Autodesk Inventor part; units mm, degrees
(part 3 of 5)
sketch "Block4" plane through (0, 0, 0) normal (0, 0, 1) x (1, 0, 0)
  line L0 (2.525, -1.7375) -> (2.525, 11.2625)
  line L1 (16.525, -1.7375) -> (16.525, 11.2625)
  line L2 (3.025, -2.2375) -> (16.025, -2.2375)
  line L3 (3.025, 11.7625) -> (16.025, 11.7625)
  arc A0 (2.525, -1.7375) -> (3.025, -2.2375) centre (3.025, -1.7375) ccw
  arc A1 (3.025, 11.7625) -> (2.525, 11.2625) centre (3.025, 11.2625) ccw
  arc A2 (16.025, -2.2375) -> (16.525, -1.7375) centre (16.025, -1.7375) ccw
  arc A3 (16.525, 11.2625) -> (16.025, 11.7625) centre (16.025, 11.2625) ccw
  line L4 (2.525, 36.3625) -> (2.525, 49.3625)
  line L5 (16.525, 36.3625) -> (16.525, 49.3625)
  line L6 (3.025, 35.8625) -> (16.025, 35.8625)
  line L7 (3.025, 49.8625) -> (16.025, 49.8625)
  arc A4 (2.525, 36.3625) -> (3.025, 35.8625) centre (3.025, 36.3625) ccw
  arc A5 (3.025, 49.8625) -> (2.525, 49.3625) centre (3.025, 49.3625) ccw
  arc A6 (16.025, 35.8625) -> (16.525, 36.3625) centre (16.025, 36.3625) ccw
  arc A7 (16.525, 49.3625) -> (16.025, 49.8625) centre (16.025, 49.3625) ccw
  line L8 (2.525, 55.4125) -> (2.525, 68.4125)
  line L9 (16.525, 55.4125) -> (16.525, 68.4125)
  line L10 (3.025, 54.9125) -> (16.025, 54.9125)
  line L11 (3.025, 68.9125) -> (16.025, 68.9125)
  arc A8 (2.525, 55.4125) -> (3.025, 54.9125) centre (3.025, 55.4125) ccw
  arc A9 (3.025, 68.9125) -> (2.525, 68.4125) centre (3.025, 68.4125) ccw
  arc A10 (16.025, 54.9125) -> (16.525, 55.4125) centre (16.025, 55.4125) ccw
  arc A11 (16.525, 68.4125) -> (16.025, 68.9125) centre (16.025, 68.4125) ccw
  line L12 (2.525, 74.4625) -> (2.525, 87.4625)
  line L13 (16.525, 74.4625) -> (16.525, 87.4625)
  line L14 (3.025, 73.9625) -> (16.025, 73.9625)
  line L15 (3.025, 87.9625) -> (16.025, 87.9625)
  arc A12 (2.525, 74.4625) -> (3.025, 73.9625) centre (3.025, 74.4625) ccw
  arc A13 (3.025, 87.9625) -> (2.525, 87.4625) centre (3.025, 87.4625) ccw
  arc A14 (16.025, 73.9625) -> (16.525, 74.4625) centre (16.025, 74.4625) ccw
  arc A15 (16.525, 87.4625) -> (16.025, 87.9625) centre (16.025, 87.4625) ccw
  line L16 (2.525, 93.5125) -> (2.525, 106.5125)
  line L17 (16.525, 93.5125) -> (16.525, 106.5125)
  line L18 (3.025, 93.0125) -> (16.025, 93.0125)
  line L19 (3.025, 107.0125) -> (16.025, 107.0125)
  arc A16 (2.525, 93.5125) -> (3.025, 93.0125) centre (3.025, 93.5125) ccw
  arc A17 (3.025, 107.0125) -> (2.525, 106.5125) centre (3.025, 106.5125) ccw
  arc A18 (16.025, 93.0125) -> (16.525, 93.5125) centre (16.025, 93.5125) ccw
  arc A19 (16.525, 106.5125) -> (16.025, 107.0125) centre (16.025, 106.5125) ccw
  line L20 (2.525, 122.0875) -> (2.525, 135.0875)
  line L21 (16.525, 122.0875) -> (16.525, 135.0875)
  line L22 (3.025, 121.5875) -> (16.025, 121.5875)
  line L23 (3.025, 135.5875) -> (16.025, 135.5875)
  arc A20 (2.525, 122.0875) -> (3.025, 121.5875) centre (3.025, 122.0875) ccw
  arc A21 (3.025, 135.5875) -> (2.525, 135.0875) centre (3.025, 135.0875) ccw
  arc A22 (16.025, 121.5875) -> (16.525, 122.0875) centre (16.025, 122.0875) ccw
  arc A23 (16.525, 135.0875) -> (16.025, 135.5875) centre (16.025, 135.0875) ccw
  line L24 (2.525, 141.1375) -> (2.525, 154.1375)
  line L25 (16.525, 141.1375) -> (16.525, 154.1375)
  line L26 (3.025, 140.6375) -> (16.025, 140.6375)
  line L27 (3.025, 154.6375) -> (16.025, 154.6375)
  arc A24 (2.525, 141.1375) -> (3.025, 140.6375) centre (3.025, 141.1375) ccw
  arc A25 (3.025, 154.6375) -> (2.525, 154.1375) centre (3.025, 154.1375) ccw
  arc A26 (16.025, 140.6375) -> (16.525, 141.1375) centre (16.025, 141.1375) ccw
  arc A27 (16.525, 154.1375) -> (16.025, 154.6375) centre (16.025, 154.1375) ccw
  line L28 (2.525, 160.1875) -> (2.525, 173.1875)
  line L29 (16.525, 160.1875) -> (16.525, 173.1875)
  line L30 (3.025, 159.6875) -> (16.025, 159.6875)
  line L31 (3.025, 173.6875) -> (16.025, 173.6875)
  arc A28 (2.525, 160.1875) -> (3.025, 159.6875) centre (3.025, 160.1875) ccw
  arc A29 (3.025, 173.6875) -> (2.525, 173.1875) centre (3.025, 173.1875) ccw
  arc A30 (16.025, 159.6875) -> (16.525, 160.1875) centre (16.025, 160.1875) ccw
  arc A31 (16.525, 173.1875) -> (16.025, 173.6875) centre (16.025, 173.1875) ccw
  line L32 (2.525, 179.2375) -> (2.525, 192.2375)
  line L33 (16.525, 179.2375) -> (16.525, 192.2375)
  line L34 (3.025, 178.7375) -> (16.025, 178.7375)
  line L35 (3.025, 192.7375) -> (16.025, 192.7375)
  arc A32 (2.525, 179.2375) -> (3.025, 178.7375) centre (3.025, 179.2375) ccw
  arc A33 (3.025, 192.7375) -> (2.525, 192.2375) centre (3.025, 192.2375) ccw
  arc A34 (16.025, 178.7375) -> (16.525, 179.2375) centre (16.025, 179.2375) ccw
  arc A35 (16.525, 192.2375) -> (16.025, 192.7375) centre (16.025, 192.2375) ccw
  line L36 (2.525, 207.8125) -> (2.525, 220.8125)
  line L37 (16.525, 207.8125) -> (16.525, 220.8125)
  line L38 (3.025, 207.3125) -> (16.025, 207.3125)
  line L39 (3.025, 221.3125) -> (16.025, 221.3125)
  arc A36 (2.525, 207.8125) -> (3.025, 207.3125) centre (3.025, 207.8125) ccw
  arc A37 (3.025, 221.3125) -> (2.525, 220.8125) centre (3.025, 220.8125) ccw
  arc A38 (16.025, 207.3125) -> (16.525, 207.8125) centre (16.025, 207.8125) ccw
  arc A39 (16.525, 220.8125) -> (16.025, 221.3125) centre (16.025, 220.8125) ccw
  line L40 (2.525, 226.8625) -> (2.525, 239.8625)
  line L41 (16.525, 226.8625) -> (16.525, 239.8625)
  line L42 (3.025, 226.3625) -> (16.025, 226.3625)
  line L43 (3.025, 240.3625) -> (16.025, 240.3625)
  arc A40 (2.525, 226.8625) -> (3.025, 226.3625) centre (3.025, 226.8625) ccw
  arc A41 (3.025, 240.3625) -> (2.525, 239.8625) centre (3.025, 239.8625) ccw
  arc A42 (16.025, 226.3625) -> (16.525, 226.8625) centre (16.025, 226.8625) ccw
  arc A43 (16.525, 239.8625) -> (16.025, 240.3625) centre (16.025, 239.8625) ccw
  line L44 (2.525, 245.9125) -> (2.525, 258.9125)
  line L45 (16.525, 245.9125) -> (16.525, 258.9125)
  line L46 (3.025, 245.4125) -> (16.025, 245.4125)
  line L47 (3.025, 259.4125) -> (16.025, 259.4125)
  arc A44 (2.525, 245.9125) -> (3.025, 245.4125) centre (3.025, 245.9125) ccw
  arc A45 (3.025, 259.4125) -> (2.525, 258.9125) centre (3.025, 258.9125) ccw
  arc A46 (16.025, 245.4125) -> (16.525, 245.9125) centre (16.025, 245.9125) ccw
  arc A47 (16.525, 258.9125) -> (16.025, 259.4125) centre (16.025, 258.9125) ccw
  line L48 (2.525, 264.9625) -> (2.525, 277.9625)
  line L49 (16.525, 264.9625) -> (16.525, 277.9625)
  line L50 (3.025, 264.4625) -> (16.025, 264.4625)
  line L51 (3.025, 278.4625) -> (16.025, 278.4625)
  arc A48 (2.525, 264.9625) -> (3.025, 264.4625) centre (3.025, 264.9625) ccw
  arc A49 (3.025, 278.4625) -> (2.525, 277.9625) centre (3.025, 277.9625) ccw
  arc A50 (16.025, 264.4625) -> (16.525, 264.9625) centre (16.025, 264.9625) ccw
  arc A51 (16.525, 277.9625) -> (16.025, 278.4625) centre (16.025, 277.9625) ccw
  line L52 (26.3375, -1.7375) -> (26.3375, 11.2625)
  line L53 (40.3375, -1.7375) -> (40.3375, 11.2625)
  line L54 (26.8375, -2.2375) -> (39.8375, -2.2375)
  line L55 (26.8375, 11.7625) -> (39.8375, 11.7625)
  arc A52 (26.3375, -1.7375) -> (26.8375, -2.2375) centre (26.8375, -1.7375) ccw
  arc A53 (26.8375, 11.7625) -> (26.3375, 11.2625) centre (26.8375, 11.2625) ccw
  arc A54 (39.8375, -2.2375) -> (40.3375, -1.7375) centre (39.8375, -1.7375) ccw
  arc A55 (40.3375, 11.2625) -> (39.8375, 11.7625) centre (39.8375, 11.2625) ccw
  line L56 (26.3375, 17.3125) -> (26.3375, 30.3125)
  line L57 (40.3375, 17.3125) -> (40.3375, 30.3125)
  line L58 (26.8375, 16.8125) -> (39.8375, 16.8125)
  line L59 (26.8375, 30.8125) -> (39.8375, 30.8125)
  arc A56 (26.3375, 17.3125) -> (26.8375, 16.8125) centre (26.8375, 17.3125) ccw
  arc A57 (26.8375, 30.8125) -> (26.3375, 30.3125) centre (26.8375, 30.3125) ccw
  arc A58 (39.8375, 16.8125) -> (40.3375, 17.3125) centre (39.8375, 17.3125) ccw
  arc A59 (40.3375, 30.3125) -> (39.8375, 30.8125) centre (39.8375, 30.3125) ccw
  line L60 (26.3375, 36.3625) -> (26.3375, 49.3625)
  line L61 (40.3375, 36.3625) -> (40.3375, 49.3625)
  line L62 (26.8375, 35.8625) -> (39.8375, 35.8625)
  line L63 (26.8375, 49.8625) -> (39.8375, 49.8625)
  arc A60 (26.3375, 36.3625) -> (26.8375, 35.8625) centre (26.8375, 36.3625) ccw
  arc A61 (26.8375, 49.8625) -> (26.3375, 49.3625) centre (26.8375, 49.3625) ccw
  arc A62 (39.8375, 35.8625) -> (40.3375, 36.3625) centre (39.8375, 36.3625) ccw
  arc A63 (40.3375, 49.3625) -> (39.8375, 49.8625) centre (39.8375, 49.3625) ccw
  line L64 (26.3375, 55.4125) -> (26.3375, 68.4125)
  line L65 (40.3375, 55.4125) -> (40.3375, 68.4125)
  line L66 (26.8375, 54.9125) -> (39.8375, 54.9125)
  line L67 (26.8375, 68.9125) -> (39.8375, 68.9125)
  arc A64 (26.3375, 55.4125) -> (26.8375, 54.9125) centre (26.8375, 55.4125) ccw
  arc A65 (26.8375, 68.9125) -> (26.3375, 68.4125) centre (26.8375, 68.4125) ccw
  arc A66 (39.8375, 54.9125) -> (40.3375, 55.4125) centre (39.8375, 55.4125) ccw
  arc A67 (40.3375, 68.4125) -> (39.8375, 68.9125) centre (39.8375, 68.4125) ccw
  line L68 (26.3375, 74.4625) -> (26.3375, 87.4625)
  line L69 (40.3375, 74.4625) -> (40.3375, 87.4625)
  line L70 (26.8375, 73.9625) -> (39.8375, 73.9625)
  line L71 (26.8375, 87.9625) -> (39.8375, 87.9625)
  arc A68 (26.3375, 74.4625) -> (26.8375, 73.9625) centre (26.8375, 74.4625) ccw
  arc A69 (26.8375, 87.9625) -> (26.3375, 87.4625) centre (26.8375, 87.4625) ccw
  arc A70 (39.8375, 73.9625) -> (40.3375, 74.4625) centre (39.8375, 74.4625) ccw
  arc A71 (40.3375, 87.4625) -> (39.8375, 87.9625) centre (39.8375, 87.4625) ccw
  line L72 (26.3375, 93.5125) -> (26.3375, 106.5125)
  line L73 (40.3375, 93.5125) -> (40.3375, 106.5125)
  line L74 (26.8375, 93.0125) -> (39.8375, 93.0125)
  line L75 (26.8375, 107.0125) -> (39.8375, 107.0125)
  arc A72 (26.3375, 93.5125) -> (26.8375, 93.0125) centre (26.8375, 93.5125) ccw
  arc A73 (26.8375, 107.0125) -> (26.3375, 106.5125) centre (26.8375, 106.5125) ccw
  arc A74 (39.8375, 93.0125) -> (40.3375, 93.5125) centre (39.8375, 93.5125) ccw
  arc A75 (40.3375, 106.5125) -> (39.8375, 107.0125) centre (39.8375, 106.5125) ccw
  line L76 (26.3375, 112.5625) -> (26.3375, 125.5625)
  line L77 (40.3375, 112.5625) -> (40.3375, 125.5625)
  line L78 (26.8375, 112.0625) -> (39.8375, 112.0625)
  line L79 (26.8375, 126.0625) -> (39.8375, 126.0625)
  arc A76 (26.3375, 112.5625) -> (26.8375, 112.0625) centre (26.8375, 112.5625) ccw
  arc A77 (26.8375, 126.0625) -> (26.3375, 125.5625) centre (26.8375, 125.5625) ccw
  arc A78 (39.8375, 112.0625) -> (40.3375, 112.5625) centre (39.8375, 112.5625) ccw
  arc A79 (40.3375, 125.5625) -> (39.8375, 126.0625) centre (39.8375, 125.5625) ccw
  line L80 (26.3375, 131.6125) -> (26.3375, 144.6125)
  line L81 (40.3375, 131.6125) -> (40.3375, 144.6125)
  line L82 (26.8375, 131.1125) -> (39.8375, 131.1125)
  line L83 (26.8375, 145.1125) -> (39.8375, 145.1125)
  arc A80 (26.3375, 131.6125) -> (26.8375, 131.1125) centre (26.8375, 131.6125) ccw
  arc A81 (26.8375, 145.1125) -> (26.3375, 144.6125) centre (26.8375, 144.6125) ccw
  arc A82 (39.8375, 131.1125) -> (40.3375, 131.6125) centre (39.8375, 131.6125) ccw
  arc A83 (40.3375, 144.6125) -> (39.8375, 145.1125) centre (39.8375, 144.6125) ccw
  line L84 (26.3375, 150.6625) -> (26.3375, 163.6625)
  line L85 (40.3375, 150.6625) -> (40.3375, 163.6625)
  line L86 (26.8375, 150.1625) -> (39.8375, 150.1625)
  line L87 (26.8375, 164.1625) -> (39.8375, 164.1625)
  arc A84 (26.3375, 150.6625) -> (26.8375, 150.1625) centre (26.8375, 150.6625) ccw
  arc A85 (26.8375, 164.1625) -> (26.3375, 163.6625) centre (26.8375, 163.6625) ccw
  arc A86 (39.8375, 150.1625) -> (40.3375, 150.6625) centre (39.8375, 150.6625) ccw
  arc A87 (40.3375, 163.6625) -> (39.8375, 164.1625) centre (39.8375, 163.6625) ccw
  line L88 (26.3375, 169.7125) -> (26.3375, 182.7125)
  line L89 (40.3375, 169.7125) -> (40.3375, 182.7125)
  line L90 (26.8375, 169.2125) -> (39.8375, 169.2125)
  line L91 (26.8375, 183.2125) -> (39.8375, 183.2125)
  arc A88 (26.3375, 169.7125) -> (26.8375, 169.2125) centre (26.8375, 169.7125) ccw
  arc A89 (26.8375, 183.2125) -> (26.3375, 182.7125) centre (26.8375, 182.7125) ccw
  arc A90 (39.8375, 169.2125) -> (40.3375, 169.7125) centre (39.8375, 169.7125) ccw
  arc A91 (40.3375, 182.7125) -> (39.8375, 183.2125) centre (39.8375, 182.7125) ccw
  line L92 (26.3375, 188.7625) -> (26.3375, 201.7625)
  line L93 (40.3375, 188.7625) -> (40.3375, 201.7625)
  line L94 (26.8375, 188.2625) -> (39.8375, 188.2625)
  line L95 (26.8375, 202.2625) -> (39.8375, 202.2625)
  arc A92 (26.3375, 188.7625) -> (26.8375, 188.2625) centre (26.8375, 188.7625) ccw
  arc A93 (26.8375, 202.2625) -> (26.3375, 201.7625) centre (26.8375, 201.7625) ccw
  arc A94 (39.8375, 188.2625) -> (40.3375, 188.7625) centre (39.8375, 188.7625) ccw
  arc A95 (40.3375, 201.7625) -> (39.8375, 202.2625) centre (39.8375, 201.7625) ccw
  line L96 (26.3375, 207.8125) -> (26.3375, 220.8125)
  line L97 (40.3375, 207.8125) -> (40.3375, 220.8125)
  line L98 (26.8375, 207.3125) -> (39.8375, 207.3125)
  line L99 (26.8375, 221.3125) -> (39.8375, 221.3125)
  arc A96 (26.3375, 207.8125) -> (26.8375, 207.3125) centre (26.8375, 207.8125) ccw
  arc A97 (26.8375, 221.3125) -> (26.3375, 220.8125) centre (26.8375, 220.8125) ccw
  arc A98 (39.8375, 207.3125) -> (40.3375, 207.8125) centre (39.8375, 207.8125) ccw
  arc A99 (40.3375, 220.8125) -> (39.8375, 221.3125) centre (39.8375, 220.8125) ccw
  line L100 (26.3375, 226.8625) -> (26.3375, 239.8625)
  line L101 (40.3375, 226.8625) -> (40.3375, 239.8625)
  line L102 (26.8375, 226.3625) -> (39.8375, 226.3625)
  line L103 (26.8375, 240.3625) -> (39.8375, 240.3625)
  arc A100 (26.3375, 226.8625) -> (26.8375, 226.3625) centre (26.8375, 226.8625) ccw
  arc A101 (26.8375, 240.3625) -> (26.3375, 239.8625) centre (26.8375, 239.8625) ccw
  arc A102 (39.8375, 226.3625) -> (40.3375, 226.8625) centre (39.8375, 226.8625) ccw
  arc A103 (40.3375, 239.8625) -> (39.8375, 240.3625) centre (39.8375, 239.8625) ccw
  line L104 (26.3375, 255.4375) -> (26.3375, 268.4375)
  line L105 (40.3375, 255.4375) -> (40.3375, 268.4375)
  line L106 (26.8375, 254.9375) -> (39.8375, 254.9375)
  line L107 (26.8375, 268.9375) -> (39.8375, 268.9375)
  arc A104 (26.3375, 255.4375) -> (26.8375, 254.9375) centre (26.8375, 255.4375) ccw
  arc A105 (26.8375, 268.9375) -> (26.3375, 268.4375) centre (26.8375, 268.4375) ccw
  arc A106 (39.8375, 254.9375) -> (40.3375, 255.4375) centre (39.8375, 255.4375) ccw
  arc A107 (40.3375, 268.4375) -> (39.8375, 268.9375) centre (39.8375, 268.4375) ccw
  line L108 (27.3375, 246.9995) -> (27.3375, 252.9995)
  line L109 (42.3375, 246.9995) -> (42.3375, 252.9995)
  line L110 (27.8375, 246.4995) -> (41.8375, 246.4995)
  line L111 (27.8375, 253.4995) -> (41.8375, 253.4995)
  arc A108 (27.3375, 246.9995) -> (27.8375, 246.4995) centre (27.8375, 246.9995) ccw
  arc A109 (27.8375, 253.4995) -> (27.3375, 252.9995) centre (27.8375, 252.9995) ccw
  arc A110 (41.8375, 246.4995) -> (42.3375, 246.9995) centre (41.8375, 246.9995) ccw
  arc A111 (42.3375, 252.9995) -> (41.8375, 253.4995) centre (41.8375, 252.9995) ccw
  line L112 (27.3375, 270.8755) -> (27.3375, 276.8755)
  line L113 (42.3375, 270.8755) -> (42.3375, 276.8755)
  line L114 (27.8375, 270.3755) -> (41.8375, 270.3755)
  line L115 (27.8375, 277.3755) -> (41.8375, 277.3755)
  arc A112 (27.3375, 270.8755) -> (27.8375, 270.3755) centre (27.8375, 270.8755) ccw
  arc A113 (27.8375, 277.3755) -> (27.3375, 276.8755) centre (27.8375, 276.8755) ccw
  arc A114 (41.8375, 270.3755) -> (42.3375, 270.8755) centre (41.8375, 270.8755) ccw
  arc A115 (42.3375, 276.8755) -> (41.8375, 277.3755) centre (41.8375, 276.8755) ccw
  line L116 (26.3375, 288.775) -> (26.3375, 301.775)
  line L117 (40.3375, 288.775) -> (40.3375, 301.775)
  line L118 (26.8375, 288.275) -> (39.8375, 288.275)
  line L119 (26.8375, 302.275) -> (39.8375, 302.275)
  arc A116 (26.3375, 288.775) -> (26.8375, 288.275) centre (26.8375, 288.775) ccw
  arc A117 (26.8375, 302.275) -> (26.3375, 301.775) centre (26.8375, 301.775) ccw
  arc A118 (39.8375, 288.275) -> (40.3375, 288.775) centre (39.8375, 288.775) ccw
  arc A119 (40.3375, 301.775) -> (39.8375, 302.275) centre (39.8375, 301.775) ccw
  line L120 (26.3375, 307.825) -> (26.3375, 320.825)
  line L121 (40.3375, 307.825) -> (40.3375, 320.825)
  line L122 (26.8375, 307.325) -> (39.8375, 307.325)
  line L123 (26.8375, 321.325) -> (39.8375, 321.325)
  arc A120 (26.3375, 307.825) -> (26.8375, 307.325) centre (26.8375, 307.825) ccw
  arc A121 (26.8375, 321.325) -> (26.3375, 320.825) centre (26.8375, 320.825) ccw
  arc A122 (39.8375, 307.325) -> (40.3375, 307.825) centre (39.8375, 307.825) ccw
  arc A123 (40.3375, 320.825) -> (39.8375, 321.325) centre (39.8375, 320.825) ccw
  line L124 (26.3375, 326.875) -> (26.3375, 339.875)
  line L125 (40.3375, 326.875) -> (40.3375, 339.875)
  line L126 (26.8375, 326.375) -> (39.8375, 326.375)
  line L127 (26.8375, 340.375) -> (39.8375, 340.375)
  arc A124 (26.3375, 326.875) -> (26.8375, 326.375) centre (26.8375, 326.875) ccw
  arc A125 (26.8375, 340.375) -> (26.3375, 339.875) centre (26.8375, 339.875) ccw
  arc A126 (39.8375, 326.375) -> (40.3375, 326.875) centre (39.8375, 326.875) ccw
  arc A127 (40.3375, 339.875) -> (39.8375, 340.375) centre (39.8375, 339.875) ccw
  line L128 (45.3875, 3.025) -> (45.3875, 16.025)
  line L129 (59.3875, 3.025) -> (59.3875, 16.025)
  line L130 (45.8875, 2.525) -> (58.8875, 2.525)
  line L131 (45.8875, 16.525) -> (58.8875, 16.525)
  arc A128 (45.3875, 3.025) -> (45.8875, 2.525) centre (45.8875, 3.025) ccw
  arc A129 (45.8875, 16.525) -> (45.3875, 16.025) centre (45.8875, 16.025) ccw
  arc A130 (58.8875, 2.525) -> (59.3875, 3.025) centre (58.8875, 3.025) ccw
  arc A131 (59.3875, 16.025) -> (58.8875, 16.525) centre (58.8875, 16.025) ccw
  line L132 (45.3875, 26.8375) -> (45.3875, 39.8375)
  line L133 (59.3875, 26.8375) -> (59.3875, 39.8375)
  line L134 (45.8875, 26.3375) -> (58.8875, 26.3375)
  line L135 (45.8875, 40.3375) -> (58.8875, 40.3375)
  arc A132 (45.3875, 26.8375) -> (45.8875, 26.3375) centre (45.8875, 26.8375) ccw
  arc A133 (45.8875, 40.3375) -> (45.3875, 39.8375) centre (45.8875, 39.8375) ccw
  arc A134 (58.8875, 26.3375) -> (59.3875, 26.8375) centre (58.8875, 26.8375) ccw
  arc A135 (59.3875, 39.8375) -> (58.8875, 40.3375) centre (58.8875, 39.8375) ccw
  line L136 (45.3875, 45.8875) -> (45.3875, 58.8875)
  line L137 (59.3875, 45.8875) -> (59.3875, 58.8875)
  line L138 (45.8875, 45.3875) -> (58.8875, 45.3875)
  line L139 (45.8875, 59.3875) -> (58.8875, 59.3875)
  arc A136 (45.3875, 45.8875) -> (45.8875, 45.3875) centre (45.8875, 45.8875) ccw
  arc A137 (45.8875, 59.3875) -> (45.3875, 58.8875) centre (45.8875, 58.8875) ccw
  arc A138 (58.8875, 45.3875) -> (59.3875, 45.8875) centre (58.8875, 45.8875) ccw
  arc A139 (59.3875, 58.8875) -> (58.8875, 59.3875) centre (58.8875, 58.8875) ccw
  line L140 (45.3875, 64.9375) -> (45.3875, 77.9375)
  line L141 (59.3875, 64.9375) -> (59.3875, 77.9375)
  line L142 (45.8875, 64.4375) -> (58.8875, 64.4375)
  line L143 (45.8875, 78.4375) -> (58.8875, 78.4375)
  arc A140 (45.3875, 64.9375) -> (45.8875, 64.4375) centre (45.8875, 64.9375) ccw
  arc A141 (45.8875, 78.4375) -> (45.3875, 77.9375) centre (45.8875, 77.9375) ccw
  arc A142 (58.8875, 64.4375) -> (59.3875, 64.9375) centre (58.8875, 64.9375) ccw
  arc A143 (59.3875, 77.9375) -> (58.8875, 78.4375) centre (58.8875, 77.9375) ccw
  line L144 (45.3875, 83.9875) -> (45.3875, 96.9875)
  line L145 (59.3875, 83.9875) -> (59.3875, 96.9875)
  line L146 (45.8875, 83.4875) -> (58.8875, 83.4875)
  line L147 (45.8875, 97.4875) -> (58.8875, 97.4875)
  arc A144 (45.3875, 83.9875) -> (45.8875, 83.4875) centre (45.8875, 83.9875) ccw
  arc A145 (45.8875, 97.4875) -> (45.3875, 96.9875) centre (45.8875, 96.9875) ccw
  arc A146 (58.8875, 83.4875) -> (59.3875, 83.9875) centre (58.8875, 83.9875) ccw
  arc A147 (59.3875, 96.9875) -> (58.8875, 97.4875) centre (58.8875, 96.9875) ccw
  line L148 (45.3875, 103.0375) -> (45.3875, 116.0375)
  line L149 (59.3875, 103.0375) -> (59.3875, 116.0375)
  line L150 (45.8875, 102.5375) -> (58.8875, 102.5375)
  line L151 (45.8875, 116.5375) -> (58.8875, 116.5375)
  arc A148 (45.3875, 103.0375) -> (45.8875, 102.5375) centre (45.8875, 103.0375) ccw
  arc A149 (45.8875, 116.5375) -> (45.3875, 116.0375) centre (45.8875, 116.0375) ccw
  arc A150 (58.8875, 102.5375) -> (59.3875, 103.0375) centre (58.8875, 103.0375) ccw
  arc A151 (59.3875, 116.0375) -> (58.8875, 116.5375) centre (58.8875, 116.0375) ccw
  line L152 (45.3875, 122.0875) -> (45.3875, 135.0875)
  line L153 (59.3875, 122.0875) -> (59.3875, 135.0875)
  line L154 (45.8875, 121.5875) -> (58.8875, 121.5875)
  line L155 (45.8875, 135.5875) -> (58.8875, 135.5875)
  arc A152 (45.3875, 122.0875) -> (45.8875, 121.5875) centre (45.8875, 122.0875) ccw
  arc A153 (45.8875, 135.5875) -> (45.3875, 135.0875) centre (45.8875, 135.0875) ccw
  arc A154 (58.8875, 121.5875) -> (59.3875, 122.0875) centre (58.8875, 122.0875) ccw
  arc A155 (59.3875, 135.0875) -> (58.8875, 135.5875) centre (58.8875, 135.0875) ccw
  line L156 (45.3875, 141.1375) -> (45.3875, 154.1375)
  line L157 (59.3875, 141.1375) -> (59.3875, 154.1375)
  line L158 (45.8875, 140.6375) -> (58.8875, 140.6375)
  line L159 (45.8875, 154.6375) -> (58.8875, 154.6375)
  arc A156 (45.3875, 141.1375) -> (45.8875, 140.6375) centre (45.8875, 141.1375) ccw
  arc A157 (45.8875, 154.6375) -> (45.3875, 154.1375) centre (45.8875, 154.1375) ccw
  arc A158 (58.8875, 140.6375) -> (59.3875, 141.1375) centre (58.8875, 141.1375) ccw
  arc A159 (59.3875, 154.1375) -> (58.8875, 154.6375) centre (58.8875, 154.1375) ccw
  line L160 (45.3875, 160.1875) -> (45.3875, 173.1875)
  line L161 (59.3875, 160.1875) -> (59.3875, 173.1875)
  line L162 (45.8875, 159.6875) -> (58.8875, 159.6875)
  line L163 (45.8875, 173.6875) -> (58.8875, 173.6875)
  arc A160 (45.3875, 160.1875) -> (45.8875, 159.6875) centre (45.8875, 160.1875) ccw
  arc A161 (45.8875, 173.6875) -> (45.3875, 173.1875) centre (45.8875, 173.1875) ccw
  arc A162 (58.8875, 159.6875) -> (59.3875, 160.1875) centre (58.8875, 160.1875) ccw
  arc A163 (59.3875, 173.1875) -> (58.8875, 173.6875) centre (58.8875, 173.1875) ccw
  line L164 (45.3875, 179.2375) -> (45.3875, 192.2375)
  line L165 (59.3875, 179.2375) -> (59.3875, 192.2375)
  line L166 (45.8875, 178.7375) -> (58.8875, 178.7375)
  line L167 (45.8875, 192.7375) -> (58.8875, 192.7375)
  arc A164 (45.3875, 179.2375) -> (45.8875, 178.7375) centre (45.8875, 179.2375) ccw
  arc A165 (45.8875, 192.7375) -> (45.3875, 192.2375) centre (45.8875, 192.2375) ccw
  arc A166 (58.8875, 178.7375) -> (59.3875, 179.2375) centre (58.8875, 179.2375) ccw
  arc A167 (59.3875, 192.2375) -> (58.8875, 192.7375) centre (58.8875, 192.2375) ccw
  line L168 (45.3875, 198.2875) -> (45.3875, 211.2875)
  line L169 (59.3875, 198.2875) -> (59.3875, 211.2875)
  line L170 (45.8875, 197.7875) -> (58.8875, 197.7875)
  line L171 (45.8875, 211.7875) -> (58.8875, 211.7875)
  arc A168 (45.3875, 198.2875) -> (45.8875, 197.7875) centre (45.8875, 198.2875) ccw
  arc A169 (45.8875, 211.7875) -> (45.3875, 211.2875) centre (45.8875, 211.2875) ccw
  arc A170 (58.8875, 197.7875) -> (59.3875, 198.2875) centre (58.8875, 198.2875) ccw
  arc A171 (59.3875, 211.2875) -> (58.8875, 211.7875) centre (58.8875, 211.2875) ccw
  line L172 (45.3875, 217.3375) -> (45.3875, 230.3375)
  line L173 (59.3875, 217.3375) -> (59.3875, 230.3375)
  line L174 (45.8875, 216.8375) -> (58.8875, 216.8375)
  line L175 (45.8875, 230.8375) -> (58.8875, 230.8375)
  arc A172 (45.3875, 217.3375) -> (45.8875, 216.8375) centre (45.8875, 217.3375) ccw
  arc A173 (45.8875, 230.8375) -> (45.3875, 230.3375) centre (45.8875, 230.3375) ccw
  arc A174 (58.8875, 216.8375) -> (59.3875, 217.3375) centre (58.8875, 217.3375) ccw
  arc A175 (59.3875, 230.3375) -> (58.8875, 230.8375) centre (58.8875, 230.3375) ccw
  line L176 (45.3875, 236.3875) -> (45.3875, 249.3875)
  line L177 (59.3875, 236.3875) -> (59.3875, 249.3875)
  line L178 (45.8875, 235.8875) -> (58.8875, 235.8875)
  line L179 (45.8875, 249.8875) -> (58.8875, 249.8875)
  arc A176 (45.3875, 236.3875) -> (45.8875, 235.8875) centre (45.8875, 236.3875) ccw
  arc A177 (45.8875, 249.8875) -> (45.3875, 249.3875) centre (45.8875, 249.3875) ccw
  arc A178 (58.8875, 235.8875) -> (59.3875, 236.3875) centre (58.8875, 236.3875) ccw
  arc A179 (59.3875, 249.3875) -> (58.8875, 249.8875) centre (58.8875, 249.3875) ccw
  line L180 (45.3875, 260.2) -> (45.3875, 273.2)
  line L181 (59.3875, 260.2) -> (59.3875, 273.2)
  line L182 (45.8875, 259.7) -> (58.8875, 259.7)
  line L183 (45.8875, 273.7) -> (58.8875, 273.7)
  arc A180 (45.3875, 260.2) -> (45.8875, 259.7) centre (45.8875, 260.2) ccw
  arc A181 (45.8875, 273.7) -> (45.3875, 273.2) centre (45.8875, 273.2) ccw
  arc A182 (58.8875, 259.7) -> (59.3875, 260.2) centre (58.8875, 260.2) ccw
  arc A183 (59.3875, 273.2) -> (58.8875, 273.7) centre (58.8875, 273.2) ccw
  line L184 (45.3875, 288.775) -> (45.3875, 301.775)
  line L185 (59.3875, 288.775) -> (59.3875, 301.775)
  line L186 (45.8875, 288.275) -> (58.8875, 288.275)
  line L187 (45.8875, 302.275) -> (58.8875, 302.275)
  arc A184 (45.3875, 288.775) -> (45.8875, 288.275) centre (45.8875, 288.775) ccw
  arc A185 (45.8875, 302.275) -> (45.3875, 301.775) centre (45.8875, 301.775) ccw
  arc A186 (58.8875, 288.275) -> (59.3875, 288.775) centre (58.8875, 288.775) ccw
  arc A187 (59.3875, 301.775) -> (58.8875, 302.275) centre (58.8875, 301.775) ccw
  line L188 (45.3875, 307.825) -> (45.3875, 320.825)
  line L189 (59.3875, 307.825) -> (59.3875, 320.825)
  line L190 (45.8875, 307.325) -> (58.8875, 307.325)
  line L191 (45.8875, 321.325) -> (58.8875, 321.325)
  arc A188 (45.3875, 307.825) -> (45.8875, 307.325) centre (45.8875, 307.825) ccw
  arc A189 (45.8875, 321.325) -> (45.3875, 320.825) centre (45.8875, 320.825) ccw
  arc A190 (58.8875, 307.325) -> (59.3875, 307.825) centre (58.8875, 307.825) ccw
  arc A191 (59.3875, 320.825) -> (58.8875, 321.325) centre (58.8875, 320.825) ccw
  line L192 (45.3875, 326.875) -> (45.3875, 339.875)
  line L193 (59.3875, 326.875) -> (59.3875, 339.875)
  line L194 (45.8875, 326.375) -> (58.8875, 326.375)
  line L195 (45.8875, 340.375) -> (58.8875, 340.375)
  arc A192 (45.3875, 326.875) -> (45.8875, 326.375) centre (45.8875, 326.875) ccw
  arc A193 (45.8875, 340.375) -> (45.3875, 339.875) centre (45.8875, 339.875) ccw
  arc A194 (58.8875, 326.375) -> (59.3875, 326.875) centre (58.8875, 326.875) ccw
  arc A195 (59.3875, 339.875) -> (58.8875, 340.375) centre (58.8875, 339.875) ccw
  line L196 (64.4375, 5.4062) -> (64.4375, 18.4062)
  line L197 (78.4375, 5.4063) -> (78.4375, 18.4063)
  line L198 (64.9375, 4.9063) -> (77.9375, 4.9062)
  line L199 (64.9375, 18.9063) -> (77.9375, 18.9062)
  arc A196 (64.4375, 5.4062) -> (64.9375, 4.9063) centre (64.9375, 5.4062) ccw
  arc A197 (64.9375, 18.9063) -> (64.4375, 18.4062) centre (64.9375, 18.4063) ccw
  arc A198 (77.9375, 4.9062) -> (78.4375, 5.4063) centre (77.9375, 5.4063) ccw
  arc A199 (78.4375, 18.4063) -> (77.9375, 18.9063) centre (77.9375, 18.4062) ccw
  line L200 (64.4375, 31.6) -> (64.4375, 44.6)
  line L201 (78.4375, 31.6) -> (78.4375, 44.6)
  line L202 (64.9375, 31.1) -> (77.9375, 31.1)
  line L203 (64.9375, 45.1) -> (77.9375, 45.1)
  arc A200 (64.4375, 31.6) -> (64.9375, 31.1) centre (64.9375, 31.6) ccw
  arc A201 (64.9375, 45.1) -> (64.4375, 44.6) centre (64.9375, 44.6) ccw
  arc A202 (77.9375, 31.1) -> (78.4375, 31.6) centre (77.9375, 31.6) ccw
  arc A203 (78.4375, 44.6) -> (77.9375, 45.1) centre (77.9375, 44.6) ccw
  line L204 (64.4375, 50.65) -> (64.4375, 63.65)
  line L205 (78.4375, 50.65) -> (78.4375, 63.65)
  line L206 (64.9375, 50.15) -> (77.9375, 50.15)
  line L207 (64.9375, 64.15) -> (77.9375, 64.15)
  arc A204 (64.4375, 50.65) -> (64.9375, 50.15) centre (64.9375, 50.65) ccw
  arc A205 (64.9375, 64.15) -> (64.4375, 63.65) centre (64.9375, 63.65) ccw
  arc A206 (77.9375, 50.15) -> (78.4375, 50.65) centre (77.9375, 50.65) ccw
  arc A207 (78.4375, 63.65) -> (77.9375, 64.15) centre (77.9375, 63.65) ccw
  line L208 (64.4375, 69.7) -> (64.4375, 82.7)
  line L209 (78.4375, 69.7) -> (78.4375, 82.7)
  line L210 (64.9375, 69.2) -> (77.9375, 69.2)
  line L211 (64.9375, 83.2) -> (77.9375, 83.2)
  arc A208 (64.4375, 69.7) -> (64.9375, 69.2) centre (64.9375, 69.7) ccw
  arc A209 (64.9375, 83.2) -> (64.4375, 82.7) centre (64.9375, 82.7) ccw
  arc A210 (77.9375, 69.2) -> (78.4375, 69.7) centre (77.9375, 69.7) ccw
  arc A211 (78.4375, 82.7) -> (77.9375, 83.2) centre (77.9375, 82.7) ccw
  line L212 (64.4375, 88.75) -> (64.4375, 101.75)
  line L213 (78.4375, 88.75) -> (78.4375, 101.75)
  line L214 (64.9375, 88.25) -> (77.9375, 88.25)
  line L215 (64.9375, 102.25) -> (77.9375, 102.25)
  arc A212 (64.4375, 88.75) -> (64.9375, 88.25) centre (64.9375, 88.75) ccw
  arc A213 (64.9375, 102.25) -> (64.4375, 101.75) centre (64.9375, 101.75) ccw
  arc A214 (77.9375, 88.25) -> (78.4375, 88.75) centre (77.9375, 88.75) ccw
  arc A215 (78.4375, 101.75) -> (77.9375, 102.25) centre (77.9375, 101.75) ccw
  line L216 (64.4375, 107.8) -> (64.4375, 120.8)
  line L217 (78.4375, 107.8) -> (78.4375, 120.8)
  line L218 (64.9375, 107.3) -> (77.9375, 107.3)
  line L219 (64.9375, 121.3) -> (77.9375, 121.3)
  arc A216 (64.4375, 107.8) -> (64.9375, 107.3) centre (64.9375, 107.8) ccw
  arc A217 (64.9375, 121.3) -> (64.4375, 120.8) centre (64.9375, 120.8) ccw
  arc A218 (77.9375, 107.3) -> (78.4375, 107.8) centre (77.9375, 107.8) ccw
  arc A219 (78.4375, 120.8) -> (77.9375, 121.3) centre (77.9375, 120.8) ccw
  line L220 (64.4375, 126.85) -> (64.4375, 139.85)
  line L221 (78.4375, 126.85) -> (78.4375, 139.85)
  line L222 (64.9375, 126.35) -> (77.9375, 126.35)
  line L223 (64.9375, 140.35) -> (77.9375, 140.35)
  arc A220 (64.4375, 126.85) -> (64.9375, 126.35) centre (64.9375, 126.85) ccw
  arc A221 (64.9375, 140.35) -> (64.4375, 139.85) centre (64.9375, 139.85) ccw
  arc A222 (77.9375, 126.35) -> (78.4375, 126.85) centre (77.9375, 126.85) ccw
  arc A223 (78.4375, 139.85) -> (77.9375, 140.35) centre (77.9375, 139.85) ccw
  line L224 (64.4375, 145.9) -> (64.4375, 158.9)
  line L225 (78.4375, 145.9) -> (78.4375, 158.9)
  line L226 (64.9375, 145.4) -> (77.9375, 145.4)
  line L227 (64.9375, 159.4) -> (77.9375, 159.4)
  arc A224 (64.4375, 145.9) -> (64.9375, 145.4) centre (64.9375, 145.9) ccw
  arc A225 (64.9375, 159.4) -> (64.4375, 158.9) centre (64.9375, 158.9) ccw
  arc A226 (77.9375, 145.4) -> (78.4375, 145.9) centre (77.9375, 145.9) ccw
  arc A227 (78.4375, 158.9) -> (77.9375, 159.4) centre (77.9375, 158.9) ccw
  line L228 (64.4375, 164.95) -> (64.4375, 177.95)
  line L229 (78.4375, 164.95) -> (78.4375, 177.95)
  line L230 (64.9375, 164.45) -> (77.9375, 164.45)
  line L231 (64.9375, 178.45) -> (77.9375, 178.45)
  arc A228 (64.4375, 164.95) -> (64.9375, 164.45) centre (64.9375, 164.95) ccw
  arc A229 (64.9375, 178.45) -> (64.4375, 177.95) centre (64.9375, 177.95) ccw
  arc A230 (77.9375, 164.45) -> (78.4375, 164.95) centre (77.9375, 164.95) ccw
  arc A231 (78.4375, 177.95) -> (77.9375, 178.45) centre (77.9375, 177.95) ccw
  line L232 (64.4375, 184) -> (64.4375, 197)
  line L233 (78.4375, 184) -> (78.4375, 197)
  line L234 (64.9375, 183.5) -> (77.9375, 183.5)
  line L235 (64.9375, 197.5) -> (77.9375, 197.5)
  arc A232 (64.4375, 184) -> (64.9375, 183.5) centre (64.9375, 184) ccw
  arc A233 (64.9375, 197.5) -> (64.4375, 197) centre (64.9375, 197) ccw
  arc A234 (77.9375, 183.5) -> (78.4375, 184) centre (77.9375, 184) ccw
  arc A235 (78.4375, 197) -> (77.9375, 197.5) centre (77.9375, 197) ccw
  line L236 (64.4375, 203.05) -> (64.4375, 216.05)
  line L237 (78.4375, 203.05) -> (78.4375, 216.05)
  line L238 (64.9375, 202.55) -> (77.9375, 202.55)
  line L239 (64.9375, 216.55) -> (77.9375, 216.55)
  arc A236 (64.4375, 203.05) -> (64.9375, 202.55) centre (64.9375, 203.05) ccw
  arc A237 (64.9375, 216.55) -> (64.4375, 216.05) centre (64.9375, 216.05) ccw
  arc A238 (77.9375, 202.55) -> (78.4375, 203.05) centre (77.9375, 203.05) ccw
  arc A239 (78.4375, 216.05) -> (77.9375, 216.55) centre (77.9375, 216.05) ccw
  line L240 (64.4375, 222.1) -> (64.4375, 235.1)
  line L241 (78.4375, 222.1) -> (78.4375, 235.1)
  line L242 (64.9375, 221.6) -> (77.9375, 221.6)
  line L243 (64.9375, 235.6) -> (77.9375, 235.6)
  arc A240 (64.4375, 222.1) -> (64.9375, 221.6) centre (64.9375, 222.1) ccw
  arc A241 (64.9375, 235.6) -> (64.4375, 235.1) centre (64.9375, 235.1) ccw
  arc A242 (77.9375, 221.6) -> (78.4375, 222.1) centre (77.9375, 222.1) ccw
  arc A243 (78.4375, 235.1) -> (77.9375, 235.6) centre (77.9375, 235.1) ccw
  line L244 (64.4375, 253.0563) -> (64.4375, 266.0563)
  line L245 (78.4375, 253.0563) -> (78.4375, 266.0563)
  line L246 (64.9375, 252.5563) -> (77.9375, 252.5563)
  line L247 (64.9375, 266.5563) -> (77.9375, 266.5563)
  arc A244 (64.4375, 253.0563) -> (64.9375, 252.5563) centre (64.9375, 253.0563) ccw
  arc A245 (64.9375, 266.5563) -> (64.4375, 266.0563) centre (64.9375, 266.0563) ccw
  arc A246 (77.9375, 252.5563) -> (78.4375, 253.0563) centre (77.9375, 253.0563) ccw
  arc A247 (78.4375, 266.0563) -> (77.9375, 266.5563) centre (77.9375, 266.0563) ccw
  line L248 (65.4375, 244.6183) -> (65.4375, 250.6183)
  line L249 (80.4375, 244.6183) -> (80.4375, 250.6183)
  line L250 (65.9375, 244.1183) -> (79.9375, 244.1182)
  line L251 (65.9375, 251.1183) -> (79.9375, 251.1183)
  arc A248 (65.4375, 244.6183) -> (65.9375, 244.1183) centre (65.9375, 244.6183) ccw
  arc A249 (65.9375, 251.1182) -> (65.4375, 250.6183) centre (65.9375, 250.6182) ccw
  arc A250 (79.9375, 244.1182) -> (80.4375, 244.6183) centre (79.9375, 244.6183) ccw
  arc A251 (80.4375, 250.6183) -> (79.9375, 251.1183) centre (79.9375, 250.6183) ccw
  line L252 (65.4375, 268.4943) -> (65.4375, 274.4943)
  line L253 (80.4375, 268.4943) -> (80.4375, 274.4943)
  line L254 (65.9375, 267.9943) -> (79.9375, 267.9943)
  line L255 (65.9375, 274.9943) -> (79.9375, 274.9943)
  arc A252 (65.4375, 268.4943) -> (65.9375, 267.9943) centre (65.9375, 268.4943) ccw
  arc A253 (65.9375, 274.9943) -> (65.4375, 274.4943) centre (65.9375, 274.4943) ccw
  arc A254 (79.9375, 267.9943) -> (80.4375, 268.4943) centre (79.9375, 268.4943) ccw
  arc A255 (80.4375, 274.4943) -> (79.9375, 274.9943) centre (79.9375, 274.4943) ccw
  line L256 (83.4875, 10.1688) -> (83.4875, 23.1688)
  line L257 (97.4875, 10.1688) -> (97.4875, 23.1687)
  line L258 (83.9875, 9.6688) -> (96.9875, 9.6688)
  line L259 (83.9875, 23.6688) -> (96.9875, 23.6687)
  arc A256 (83.4875, 10.1688) -> (83.9875, 9.6688) centre (83.9875, 10.1687) ccw
  arc A257 (83.9875, 23.6688) -> (83.4875, 23.1688) centre (83.9875, 23.1688) ccw
  arc A258 (96.9875, 9.6688) -> (97.4875, 10.1688) centre (96.9875, 10.1688) ccw
  arc A259 (97.4875, 23.1687) -> (96.9875, 23.6687) centre (96.9875, 23.1687) ccw
  line L260 (84.4875, 1.7307) -> (84.4875, 7.7308)
  line L261 (99.4875, 1.7308) -> (99.4875, 7.7307)
  line L262 (84.9875, 1.2307) -> (98.9875, 1.2308)
  line L263 (84.9875, 8.2308) -> (98.9875, 8.2308)
  arc A260 (84.4875, 1.7307) -> (84.9875, 1.2307) centre (84.9875, 1.7308) ccw
  arc A261 (84.9875, 8.2308) -> (84.4875, 7.7308) centre (84.9875, 7.7308) ccw
  arc A262 (98.9875, 1.2307) -> (99.4875, 1.7308) centre (98.9875, 1.7307) ccw
  arc A263 (99.4875, 7.7307) -> (98.9875, 8.2308) centre (98.9875, 7.7308) ccw
  line L264 (84.4875, 25.6067) -> (84.4875, 31.6067)
  line L265 (99.4875, 25.6068) -> (99.4875, 31.6067)
  line L266 (84.9875, 25.1067) -> (98.9875, 25.1068)
  line L267 (84.9875, 32.1068) -> (98.9875, 32.1067)
  arc A264 (84.4875, 25.6067) -> (84.9875, 25.1068) centre (84.9875, 25.6068) ccw
  arc A265 (84.9875, 32.1068) -> (84.4875, 31.6067) centre (84.9875, 31.6068) ccw
  arc A266 (98.9875, 25.1068) -> (99.4875, 25.6067) centre (98.9875, 25.6067) ccw
  arc A267 (99.4875, 31.6067) -> (98.9875, 32.1067) centre (98.9875, 31.6067) ccw
  line L268 (83.4875, 41.125) -> (83.4875, 54.125)
  line L269 (97.4875, 41.125) -> (97.4875, 54.125)
  line L270 (83.9875, 40.625) -> (96.9875, 40.625)
  line L271 (83.9875, 54.625) -> (96.9875, 54.625)
  arc A268 (83.4875, 41.125) -> (83.9875, 40.625) centre (83.9875, 41.125) ccw
  arc A269 (83.9875, 54.625) -> (83.4875, 54.125) centre (83.9875, 54.125) ccw
  arc A270 (96.9875, 40.625) -> (97.4875, 41.125) centre (96.9875, 41.125) ccw
  arc A271 (97.4875, 54.125) -> (96.9875, 54.625) centre (96.9875, 54.125) ccw
  line L272 (83.4875, 60.175) -> (83.4875, 73.175)
  line L273 (97.4875, 60.175) -> (97.4875, 73.175)
  line L274 (83.9875, 59.675) -> (96.9875, 59.675)
  line L275 (83.9875, 73.675) -> (96.9875, 73.675)
  arc A272 (83.4875, 60.175) -> (83.9875, 59.675) centre (83.9875, 60.175) ccw
  arc A273 (83.9875, 73.675) -> (83.4875, 73.175) centre (83.9875, 73.175) ccw
  arc A274 (96.9875, 59.675) -> (97.4875, 60.175) centre (96.9875, 60.175) ccw
  arc A275 (97.4875, 73.175) -> (96.9875, 73.675) centre (96.9875, 73.175) ccw
  line L276 (83.4875, 79.225) -> (83.4875, 92.225)
  line L277 (97.4875, 79.225) -> (97.4875, 92.225)
  line L278 (83.9875, 78.725) -> (96.9875, 78.725)
  line L279 (83.9875, 92.725) -> (96.9875, 92.725)
  arc A276 (83.4875, 79.225) -> (83.9875, 78.725) centre (83.9875, 79.225) ccw
  arc A277 (83.9875, 92.725) -> (83.4875, 92.225) centre (83.9875, 92.225) ccw
  arc A278 (96.9875, 78.725) -> (97.4875, 79.225) centre (96.9875, 79.225) ccw
  arc A279 (97.4875, 92.225) -> (96.9875, 92.725) centre (96.9875, 92.225) ccw
  line L280 (83.4875, 98.275) -> (83.4875, 111.275)
  line L281 (97.4875, 98.275) -> (97.4875, 111.275)
  line L282 (83.9875, 97.775) -> (96.9875, 97.775)
  line L283 (83.9875, 111.775) -> (96.9875, 111.775)
  arc A280 (83.4875, 98.275) -> (83.9875, 97.775) centre (83.9875, 98.275) ccw
  arc A281 (83.9875, 111.775) -> (83.4875, 111.275) centre (83.9875, 111.275) ccw
  arc A282 (96.9875, 97.775) -> (97.4875, 98.275) centre (96.9875, 98.275) ccw
  arc A283 (97.4875, 111.275) -> (96.9875, 111.775) centre (96.9875, 111.275) ccw
  line L284 (83.4875, 117.325) -> (83.4875, 130.325)
  line L285 (97.4875, 117.325) -> (97.4875, 130.325)
  line L286 (83.9875, 116.825) -> (96.9875, 116.825)
  line L287 (83.9875, 130.825) -> (96.9875, 130.825)
  arc A284 (83.4875, 117.325) -> (83.9875, 116.825) centre (83.9875, 117.325) ccw
  arc A285 (83.9875, 130.825) -> (83.4875, 130.325) centre (83.9875, 130.325) ccw
  arc A286 (96.9875, 116.825) -> (97.4875, 117.325) centre (96.9875, 117.325) ccw
  arc A287 (97.4875, 130.325) -> (96.9875, 130.825) centre (96.9875, 130.325) ccw
  line L288 (83.4875, 136.375) -> (83.4875, 149.375)
  line L289 (97.4875, 136.375) -> (97.4875, 149.375)
  line L290 (83.9875, 135.875) -> (96.9875, 135.875)
  line L291 (83.9875, 149.875) -> (96.9875, 149.875)
  arc A288 (83.4875, 136.375) -> (83.9875, 135.875) centre (83.9875, 136.375) ccw
  arc A289 (83.9875, 149.875) -> (83.4875, 149.375) centre (83.9875, 149.375) ccw
  arc A290 (96.9875, 135.875) -> (97.4875, 136.375) centre (96.9875, 136.375) ccw
  arc A291 (97.4875, 149.375) -> (96.9875, 149.875) centre (96.9875, 149.375) ccw
  line L292 (83.4875, 155.425) -> (83.4875, 168.425)
  line L293 (97.4875, 155.425) -> (97.4875, 168.425)
  line L294 (83.9875, 154.925) -> (96.9875, 154.925)
  line L295 (83.9875, 168.925) -> (96.9875, 168.925)
  arc A292 (83.4875, 155.425) -> (83.9875, 154.925) centre (83.9875, 155.425) ccw
  arc A293 (83.9875, 168.925) -> (83.4875, 168.425) centre (83.9875, 168.425) ccw
  arc A294 (96.9875, 154.925) -> (97.4875, 155.425) centre (96.9875, 155.425) ccw
  arc A295 (97.4875, 168.425) -> (96.9875, 168.925) centre (96.9875, 168.425) ccw
  line L296 (83.4875, 174.475) -> (83.4875, 187.475)
  line L297 (97.4875, 174.475) -> (97.4875, 187.475)
  line L298 (83.9875, 173.975) -> (96.9875, 173.975)
  line L299 (83.9875, 187.975) -> (96.9875, 187.975)
  arc A296 (83.4875, 174.475) -> (83.9875, 173.975) centre (83.9875, 174.475) ccw
  arc A297 (83.9875, 187.975) -> (83.4875, 187.475) centre (83.9875, 187.475) ccw
  arc A298 (96.9875, 173.975) -> (97.4875, 174.475) centre (96.9875, 174.475) ccw
  arc A299 (97.4875, 187.475) -> (96.9875, 187.975) centre (96.9875, 187.475) ccw
  line L300 (83.4875, 193.525) -> (83.4875, 206.525)
  line L301 (97.4875, 193.525) -> (97.4875, 206.525)
  line L302 (83.9875, 193.025) -> (96.9875, 193.025)
  line L303 (83.9875, 207.025) -> (96.9875, 207.025)
  arc A300 (83.4875, 193.525) -> (83.9875, 193.025) centre (83.9875, 193.525) ccw
  arc A301 (83.9875, 207.025) -> (83.4875, 206.525) centre (83.9875, 206.525) ccw
  arc A302 (96.9875, 193.025) -> (97.4875, 193.525) centre (96.9875, 193.525) ccw
  arc A303 (97.4875, 206.525) -> (96.9875, 207.025) centre (96.9875, 206.525) ccw
  line L304 (83.4875, 212.575) -> (83.4875, 225.575)
  line L305 (97.4875, 212.575) -> (97.4875, 225.575)
  line L306 (83.9875, 212.075) -> (96.9875, 212.075)
  line L307 (83.9875, 226.075) -> (96.9875, 226.075)
  arc A304 (83.4875, 212.575) -> (83.9875, 212.075) centre (83.9875, 212.575) ccw
  arc A305 (83.9875, 226.075) -> (83.4875, 225.575) centre (83.9875, 225.575) ccw
  arc A306 (96.9875, 212.075) -> (97.4875, 212.575) centre (96.9875, 212.575) ccw
  arc A307 (97.4875, 225.575) -> (96.9875, 226.075) centre (96.9875, 225.575) ccw
  line L308 (83.4875, 248.2938) -> (83.4875, 261.2938)
  line L309 (97.4875, 248.2938) -> (97.4875, 261.2938)
  line L310 (83.9875, 247.7938) -> (96.9875, 247.7938)
  line L311 (83.9875, 261.7937) -> (96.9875, 261.7938)
  arc A308 (83.4875, 248.2938) -> (83.9875, 247.7938) centre (83.9875, 248.2938) ccw
  arc A309 (83.9875, 261.7938) -> (83.4875, 261.2938) centre (83.9875, 261.2938) ccw
  arc A310 (96.9875, 247.7938) -> (97.4875, 248.2938) centre (96.9875, 248.2938) ccw
  arc A311 (97.4875, 261.2938) -> (96.9875, 261.7937) centre (96.9875, 261.2938) ccw
  line L312 (84.4875, 239.8558) -> (84.4875, 245.8558)
  line L313 (99.4875, 239.8558) -> (99.4875, 245.8558)
  line L314 (84.9875, 239.3558) -> (98.9875, 239.3558)
  line L315 (84.9875, 246.3558) -> (98.9875, 246.3558)
  arc A312 (84.4875, 239.8558) -> (84.9875, 239.3558) centre (84.9875, 239.8558) ccw
  arc A313 (84.9875, 246.3558) -> (84.4875, 245.8558) centre (84.9875, 245.8558) ccw
  arc A314 (98.9875, 239.3558) -> (99.4875, 239.8558) centre (98.9875, 239.8558) ccw
  arc A315 (99.4875, 245.8558) -> (98.9875, 246.3558) centre (98.9875, 245.8558) ccw
  line L316 (84.4875, 263.7318) -> (84.4875, 269.7318)
  line L317 (99.4875, 263.7318) -> (99.4875, 269.7318)
  line L318 (84.9875, 263.2318) -> (98.9875, 263.2318)
  line L319 (84.9875, 270.2318) -> (98.9875, 270.2318)
  arc A316 (84.4875, 263.7318) -> (84.9875, 263.2318) centre (84.9875, 263.7318) ccw
  arc A317 (84.9875, 270.2318) -> (84.4875, 269.7318) centre (84.9875, 269.7318) ccw
  arc A318 (98.9875, 263.2318) -> (99.4875, 263.7318) centre (98.9875, 263.7318) ccw
  arc A319 (99.4875, 269.7318) -> (98.9875, 270.2318) centre (98.9875, 269.7318) ccw
  line L320 (83.4875, 307.825) -> (83.4875, 320.825)
  line L321 (97.4875, 307.825) -> (97.4875, 320.825)
  line L322 (83.9875, 307.325) -> (96.9875, 307.325)
  line L323 (83.9875, 321.325) -> (96.9875, 321.325)
  arc A320 (83.4875, 307.825) -> (83.9875, 307.325) centre (83.9875, 307.825) ccw
  arc A321 (83.9875, 321.325) -> (83.4875, 320.825) centre (83.9875, 320.825) ccw
  arc A322 (96.9875, 307.325) -> (97.4875, 307.825) centre (96.9875, 307.825) ccw
  arc A323 (97.4875, 320.825) -> (96.9875, 321.325) centre (96.9875, 320.825) ccw
  line L324 (102.5375, 0.6438) -> (102.5375, 13.6438)
  line L325 (116.5375, 0.6437) -> (116.5375, 13.6438)
  line L326 (103.0375, 0.1437) -> (116.0375, 0.1438)
  line L327 (103.0375, 14.1438) -> (116.0375, 14.1437)
  arc A324 (102.5375, 0.6438) -> (103.0375, 0.1437) centre (103.0375, 0.6437) ccw
  arc A325 (103.0375, 14.1438) -> (102.5375, 13.6437) centre (103.0375, 13.6438) ccw
  arc A326 (116.0375, 0.1437) -> (116.5375, 0.6437) centre (116.0375, 0.6437) ccw
  arc A327 (116.5375, 13.6438) -> (116.0375, 14.1437) centre (116.0375, 13.6437) ccw
  line L328 (102.5375, 24.4563) -> (102.5375, 37.4563)
  line L329 (116.5375, 24.4562) -> (116.5375, 37.4563)
  line L330 (103.0375, 23.9563) -> (116.0375, 23.9562)
  line L331 (103.0375, 37.9563) -> (116.0375, 37.9563)
  arc A328 (102.5375, 24.4563) -> (103.0375, 23.9563) centre (103.0375, 24.4563) ccw
  arc A329 (103.0375, 37.9563) -> (102.5375, 37.4563) centre (103.0375, 37.4562) ccw
  arc A330 (116.0375, 23.9562) -> (116.5375, 24.4562) centre (116.0375, 24.4562) ccw
  arc A331 (116.5375, 37.4563) -> (116.0375, 37.9563) centre (116.0375, 37.4562) ccw
  line L332 (102.5375, 48.2688) -> (102.5375, 61.2687)
  line L333 (116.5375, 48.2688) -> (116.5375, 61.2687)
  line L334 (103.0375, 47.7688) -> (116.0375, 47.7688)
  line L335 (103.0375, 61.7688) -> (116.0375, 61.7688)
  arc A332 (102.5375, 48.2688) -> (103.0375, 47.7688) centre (103.0375, 48.2687) ccw
  arc A333 (103.0375, 61.7688) -> (102.5375, 61.2687) centre (103.0375, 61.2688) ccw
  arc A334 (116.0375, 47.7687) -> (116.5375, 48.2688) centre (116.0375, 48.2687) ccw
  arc A335 (116.5375, 61.2687) -> (116.0375, 61.7688) centre (116.0375, 61.2688) ccw
  line L336 (102.5375, 119.7063) -> (102.5375, 132.7063)
  line L337 (116.5375, 119.7063) -> (116.5375, 132.7063)
  line L338 (103.0375, 119.2063) -> (116.0375, 119.2063)
  line L339 (103.0375, 133.2062) -> (116.0375, 133.2063)
  arc A336 (102.5375, 119.7063) -> (103.0375, 119.2063) centre (103.0375, 119.7063) ccw
  arc A337 (103.0375, 133.2062) -> (102.5375, 132.7063) centre (103.0375, 132.7062) ccw
  arc A338 (116.0375, 119.2062) -> (116.5375, 119.7063) centre (116.0375, 119.7063) ccw
  arc A339 (116.5375, 132.7063) -> (116.0375, 133.2063) centre (116.0375, 132.7063) ccw
  line L340 (103.5375, 73.2062) -> (103.5375, 79.2062)
  line L341 (118.5375, 73.2063) -> (118.5375, 79.2063)
  line L342 (104.0375, 72.7063) -> (118.0375, 72.7063)
  line L343 (104.0375, 79.7063) -> (118.0375, 79.7063)
  arc A340 (103.5375, 73.2062) -> (104.0375, 72.7062) centre (104.0375, 73.2063) ccw
  arc A341 (104.0375, 79.7063) -> (103.5375, 79.2062) centre (104.0375, 79.2063) ccw
  arc A342 (118.0375, 72.7062) -> (118.5375, 73.2063) centre (118.0375, 73.2063) ccw
  arc A343 (118.5375, 79.2063) -> (118.0375, 79.7063) centre (118.0375, 79.2063) ccw
  line L344 (103.5375, 173.2063) -> (103.5375, 179.2063)
  line L345 (118.5375, 173.2063) -> (118.5375, 179.2062)
  line L346 (104.0375, 172.7062) -> (118.0375, 172.7063)
  line L347 (104.0375, 179.7063) -> (118.0375, 179.7063)
  arc A344 (103.5375, 173.2063) -> (104.0375, 172.7062) centre (104.0375, 173.2063) ccw
  arc A345 (104.0375, 179.7063) -> (103.5375, 179.2063) centre (104.0375, 179.2063) ccw
  arc A346 (118.0375, 172.7062) -> (118.5375, 173.2063) centre (118.0375, 173.2062) ccw
  arc A347 (118.5375, 179.2063) -> (118.0375, 179.7063) centre (118.0375, 179.2063) ccw
  line L348 (102.5375, 191.1438) -> (102.5375, 204.1438)
  line L349 (116.5375, 191.1438) -> (116.5375, 204.1438)
  line L350 (103.0375, 190.6438) -> (116.0375, 190.6438)
  line L351 (103.0375, 204.6438) -> (116.0375, 204.6437)
  arc A348 (102.5375, 191.1438) -> (103.0375, 190.6438) centre (103.0375, 191.1438) ccw
  arc A349 (103.0375, 204.6438) -> (102.5375, 204.1438) centre (103.0375, 204.1438) ccw
  arc A350 (116.0375, 190.6438) -> (116.5375, 191.1438) centre (116.0375, 191.1438) ccw
  arc A351 (116.5375, 204.1438) -> (116.0375, 204.6437) centre (116.0375, 204.1438) ccw
  line L352 (102.5375, 214.9563) -> (102.5375, 227.9563)
  line L353 (116.5375, 214.9563) -> (116.5375, 227.9563)
  line L354 (103.0375, 214.4563) -> (116.0375, 214.4563)
  line L355 (103.0375, 228.4563) -> (116.0375, 228.4562)
  arc A352 (102.5375, 214.9563) -> (103.0375, 214.4563) centre (103.0375, 214.9563) ccw
  arc A353 (103.0375, 228.4563) -> (102.5375, 227.9563) centre (103.0375, 227.9563) ccw
  arc A354 (116.0375, 214.4563) -> (116.5375, 214.9563) centre (116.0375, 214.9562) ccw
  arc A355 (116.5375, 227.9563) -> (116.0375, 228.4562) centre (116.0375, 227.9562) ccw
  line L356 (102.5375, 238.7688) -> (102.5375, 251.7688)
  line L357 (116.5375, 238.7687) -> (116.5375, 251.7688)
  line L358 (103.0375, 238.2688) -> (116.0375, 238.2688)
  line L359 (103.0375, 252.2687) -> (116.0375, 252.2687)
  arc A356 (102.5375, 238.7688) -> (103.0375, 238.2688) centre (103.0375, 238.7688) ccw
  arc A357 (103.0375, 252.2687) -> (102.5375, 251.7688) centre (103.0375, 251.7688) ccw
  arc A358 (116.0375, 238.2688) -> (116.5375, 238.7687) centre (116.0375, 238.7688) ccw
  arc A359 (116.5375, 251.7688) -> (116.0375, 252.2687) centre (116.0375, 251.7688) ccw
  line L360 (102.5375, 262.5813) -> (102.5375, 275.5813)
  line L361 (116.5375, 262.5813) -> (116.5375, 275.5813)
  line L362 (103.0375, 262.0813) -> (116.0375, 262.0813)
  line L363 (103.0375, 276.0813) -> (116.0375, 276.0813)
  arc A360 (102.5375, 262.5813) -> (103.0375, 262.0812) centre (103.0375, 262.5813) ccw
  arc A361 (103.0375, 276.0813) -> (102.5375, 275.5813) centre (103.0375, 275.5812) ccw
  arc A362 (116.0375, 262.0813) -> (116.5375, 262.5812) centre (116.0375, 262.5813) ccw
  arc A363 (116.5375, 275.5813) -> (116.0375, 276.0813) centre (116.0375, 275.5813) ccw
  line L364 (102.5375, 288.775) -> (102.5375, 301.775)
  line L365 (116.5375, 288.775) -> (116.5375, 301.775)
  line L366 (103.0375, 288.275) -> (116.0375, 288.275)
  line L367 (103.0375, 302.275) -> (116.0375, 302.275)
  arc A364 (102.5375, 288.775) -> (103.0375, 288.275) centre (103.0375, 288.775) ccw
  arc A365 (103.0375, 302.275) -> (102.5375, 301.775) centre (103.0375, 301.775) ccw
  arc A366 (116.0375, 288.275) -> (116.5375, 288.775) centre (116.0375, 288.775) ccw
  arc A367 (116.5375, 301.775) -> (116.0375, 302.275) centre (116.0375, 301.775) ccw
  line L368 (102.5375, 307.825) -> (102.5375, 320.825)
  line L369 (116.5375, 307.825) -> (116.5375, 320.825)
  line L370 (103.0375, 307.325) -> (116.0375, 307.325)
  line L371 (103.0375, 321.325) -> (116.0375, 321.325)
  arc A368 (102.5375, 307.825) -> (103.0375, 307.325) centre (103.0375, 307.825) ccw
  arc A369 (103.0375, 321.325) -> (102.5375, 320.825) centre (103.0375, 320.825) ccw